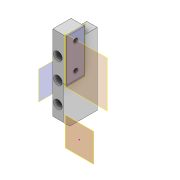
# Autodesk Inventor part: 30_XYTable_Aliexpress_Translatorarm_x
Saved by Autodesk Inventor 2022 (Build 260153000, 153)
## iProperties
Created: 2022-10-26
Part Number: 30_XYTable_Aliexpress_Translatorarm_x
Material: Generisch
Document SubType Name: Modeling
Designer: diederichbenedict
Density: 1 g/cm^3
Appearance: Vorgabe
Author: diederichbenedict
Autodesk Inventor part; units mm, degrees
ref_plane "YZ Plane" through (0, 0, 0) normal (1, 0, 0) x (0, 1, 0)
ref_plane "XZ Plane" through (0, 0, 0) normal (0, 1, 0) x (-1, 0, 0)
ref_plane "XY Plane" through (0, 0, 0) normal (0, 0, 1) x (1, 0, 0)
ref_plane "Arbeitsebene1" through (0, 0, 0) normal (0, 0, 1) x (1, 0, 0)
ref_plane "Arbeitsebene2" through (-25.4, 26.0506, 0) normal (-1, 0, 0) x (0, 0, 1)
sketch "Skizze2" plane through (-25.4, 26.0506, 0) normal (-1, 0, 0) x (0, 0, 1)
  line L0 (0, 0) -> (0, 32.2) projected
  line L1 (0, 24.2) -> (-26, 24.2)
  line L2 (-26, 24.2) -> (-26, -30.8)
  line L3 (-26, -30.8) -> (0, -30.8)
  line L4 (0, -30.8) -> (0, 24.2)
  line L5 (5, 0) -> (0, 0)
  line L6 (0, 0) -> (0, -30.8)
  line L7 (0, -30.8) -> (5, -30.8)
  point P0 (0, -26.0506)
  dimension "d26" = 26
  dimension "d27" = 55
  constraints: 14 end point, 3 parallel, 2 horizontal, 2 perpendicular, 1 point on line
  measures "d26" distance of L3.end L2.end
  measures "d27" distance of L2.end L1.end
extrude "Extrusion2" add sketch "Skizze2" against normal blind 8
ref_plane "Arbeitsebene3" through (0, 0, 5) normal (0, 0, 1) x (1, 0, 0)
sketch "Skizze6" plane through (0, 0, 5) normal (0, 0, 1) x (1, 0, 0)
  point P0 (0, 0)
ref_plane "Arbeitsebene4" through (0, 0, 5) normal (0, 0, 1) x (1, 0, 0)
ref_plane "Arbeitsebene5" through (-15, 26.0506, 0) normal (-1, 0, 0) x (0, 0, 1)
sketch "Skizze8" plane through (-15, 26.0506, 0) normal (-1, 0, 0) x (0, 0, 1)
  line L0 (-14, 32.2) -> (-14, 0) projected
  line L1 (0, 0) -> (-14, 0) projected
  line L2 (0, 32.2) -> (0, 0) projected
  line L3 (0, 32.2) -> (-14, 32.2) projected
  line L4 (-8.5, 27.35) -> (0, 27.35)
  line L5 (-8.5, 24.85) -> (0, 24.85)
  line L6 (-8.5, 7.35) -> (0, 7.35)
  line L7 (-8.5, 4.85) -> (0, 4.85)
  circle A0 centre (-7, 26.15) radius 1.6
  circle A1 centre (-7, 6.15) radius 1.6
  point P0 (0, -26.0506)
  dimension "d44" = 3.2
  dimension "d45" = 3.2
  dimension "d46" = 1.2
  dimension "d47" = 1.2
  constraints: 8 end point, 4 horizontal, 2 centre point, 8 other
  measures "d44" diameter of A0
  measures "d45" diameter of A1
  measures "d46" distance from line of A0.centre L4
  measures "d47" distance from line of L6 A1.centre
extrude "Extrusion6" add sketch "Skizze8" along normal up to surface (10.4 mm away) contours L3 L2 L4 A0 L5 L6 A1 L7 L1 L0 | L2 L5 A0 L4 | L7 A1 L6 L2
sketch "Skizze9" plane through (-25.4, 26.0506, 0) normal (-1, 0, 0) x (0, 0, 1)
  circle A0 centre (-7, 6.15) radius 1.6 projected
  circle A1 centre (-7, 26.15) radius 1.6 projected
  point P0 (0, -26.0506)
hole "Bohrung2" at (-25.4, 32.2006, -7) at (-25.4, 52.2006, -7) direction (1, 0, 0) diameter 3.2 end through all counterbore diameter 6.5 counterbore depth 5
sketch "Skizze7" plane through (0, 0, 5) normal (0, 0, 1) x (1, 0, 0)
  line L0 (15, 26.0506) -> (15, 58.2506) projected
  line L1 (15, 58.2506) -> (-25.4, 58.2506) projected
  line L2 (-25.4, 58.2506) -> (-25.4, -4.7494) projected
  line L3 (-25.4, -4.7494) -> (-17.4, -4.7494) projected
  line L4 (-17.4, 26.0506) -> (-17.4, -4.7494) projected
  line L5 (-17.4, 26.0506) -> (15, 26.0506) projected
  circle A0 centre (-21.4, 10.1506) radius 1.5
  circle A1 centre (-21.4, 26.1506) radius 1.4
  circle A2 centre (-21.4, 42.1506) radius 1.4
  point P0 (0, 0)
  dimension "d38" = 3
  dimension "d57" = 2.8
  dimension "d58" = 2.8
  dimension "d59" = 16
  dimension "d60" = 16
  dimension "d61" = 8
  dimension "d62" = 4
  dimension "d63" = 4
  dimension "d64" = 4
  dimension "d65" = 16.1
  constraints: 3 centre point
  measures "d38" diameter of A0
  measures "d57" diameter of A1
  measures "d58" diameter of A2
  measures "d59" distance of A1.centre A0.centre
  measures "d60" distance of A2.centre A1.centre
  measures "d61" distance between parallel lines of L2 L4
  measures "d62" distance from line of L4 A0.centre
  measures "d63" distance from line of A1.centre L4
  measures "d64" distance from line of A2.centre L4
  measures "d65" distance from line of A2.centre L5
hole "Bohrung1" at (-21.4, 42.1506, 5) at (-21.4, 26.1506, 5) at (-21.4, 10.1506, 5) direction (0, 0, -1) diameter 3.2 end through all counterbore diameter 6.5 counterbore depth 20
sketch "Skizze10" plane through (-15, 26.0506, 0) normal (1, 0, 0) x (0, 0, -1)
  line L0 (0, 32.2) -> (14, 32.2)
  line L1 (14, 0) -> (14, 32.2)
  line L2 (0, 0) -> (0, 32.2)
  circle A0 centre (-2.5, 50.2) radius 1.5 construction
  circle A1 centre (12.5, 50.2) radius 1.5 construction
  line L3 (13, 67.2) -> (-3, 67.2)
  line L4 (-5, 66.0453) -> (-5, 48.3547)
  line L5 (14.75, 176.5265) -> (14.75, -9.4735)
  line L6 (-5, 32.2) -> (14.75, 32.2)
  line L7 (14.75, 32.2) -> (14.75, 67.2)
  line L8 (14.75, 67.2) -> (-5, 67.2)
  line L9 (-5, 67.2) -> (-5, 32.2)
  line L10 (10, 52.2) -> (10, 45.2)
  line L11 (10, 52.2) -> (8.35, 52.2)
  line L12 (0, 45.2) -> (0, 52.2)
  line L13 (10, 44.2036) -> (0, 44.2036)
  line L14 (0, 44.2036) -> (0, 57.2)
  line L15 (0, 57.2) -> (10, 57.2)
  line L16 (10, 57.2) -> (10, 44.2036)
  circle A2 centre (12.5, 50.2) radius 1.4
  circle A3 centre (-2.5, 50.2) radius 1.4
  line L17 (-5, 32.2) -> (0, 27.2)
  line L18 (0, -30.8) -> (0, 32.2) projected
  line L19 (-5, 32.2) -> (2.0711, 32.2) construction
  line L20 (0, 27.2) -> (0, 32.2)
  line L21 (14.75, 32.2) -> (14.75, 24.2)
  line L22 (26, 24.2) -> (14, 24.2) projected
  point P0 (0, -26.0506)
  point P1 (10, 45.2)
  point P2 (0, 32.2)
  point P3 (14.75, 32.2)
  point P4 (13, 67.2)
  point P5 (0, 27.2)
  dimension "d66" = 2.8
  dimension "d67" = 2.8
  dimension "d70" = 45
  constraints: 42 end point, 6 horizontal, 6 vertical, 4 centre point, 4 parallel, 4 point on line, 2 coincident, 2 perpendicular, 1 collinear, 1 equal length, 19 other
  measures "d66" diameter of A2
  measures "d67" diameter of A3
  measures "d70" angle of L17 L19
extrude "Extrusion7" [suppressed]
chamfer "Fase2" distance 5 angle 45 1 edges at (-21.4, -4.7494, 0)
